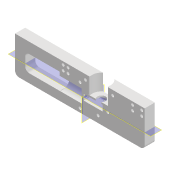
# Autodesk Inventor part: 10_Wellplate_base_p2_v1
Saved by Autodesk Inventor 2022 (Build 260153000, 153)
## iProperties
Created: 2022-04-18
Part Number: 10_Wellplate_base_p2_v1
Material: Generic
Document SubType Name: Modeling
Designer: Prakash Lab
Density: 1 g/cm^3
Appearance: Default
Author: Prakash Lab
Autodesk Inventor part; units mm, degrees
ref_plane "YZ Plane" through (0, 0, 0) normal (1, 0, 0) x (0, 1, 0)
ref_plane "XZ Plane" through (0, 0, 0) normal (0, 1, 0) x (-1, 0, 0)
ref_plane "XY Plane" through (0, 0, 0) normal (0, 0, 1) x (1, 0, 0)
sketch "Sketch1" plane through (0, 0, 0) normal (0, 0, 1) x (1, 0, 0)
  line L0 (63.9, -42.75) -> (-63.9, -42.75)
  line L1 (-63.9, -42.75) -> (-63.9, 0)
  line L2 (-63.9, 0) -> (63.9, 0)
  line L3 (63.9, 0) -> (63.9, -42.75)
  point P0 (0, 0)
  dimension "d0" = 127.8
  dimension "d178" = 63.9
  dimension "d179" = 0
  constraints: 8 end point, 2 parallel, 1 horizontal, 1 perpendicular
  measures "d0" distance of L0.start L0.end
  measures "d178" distance from line of point (0, 0) L1
  measures "d179" distance from line of L2 point (0, 0)
extrude "Extrusion1" add sketch "Sketch1" along normal blind 10
fillet "Fillet1" radius 4 4 edges at (63.9, 0, 5) (-63.9, 0, 5) (-63.9, -42.75, 5) (63.9, -42.75, 5)
sketch "Skizze38" plane through (0, 0, 10) normal (0, 0, 1) x (1, 0, 0)
  line L0 (-63.9, -4) -> (-63.9, -38.75) projected
  arc A0 (-63.9, -38.75) -> (-59.9, -42.75) centre (-59.9, -38.75) ccw projected
  line L1 (-59.9, -42.75) -> (59.9, -42.75) projected
  arc A1 (59.9, -42.75) -> (63.9, -38.75) centre (59.9, -38.75) ccw projected
  line L2 (63.9, -38.75) -> (63.9, -4) projected
  arc A2 (63.9, -4) -> (59.9, 0) centre (59.9, -4) ccw projected
  line L3 (59.9, 0) -> (-59.9, 0) projected
  arc A3 (-59.9, 0) -> (-63.9, -4) centre (-59.9, -4) ccw projected
  point P0 (0, 0)
  point P1 (9.5347, -23.74)
  point P2 (0.0978, -16.7743)
  point P3 (0.0978, -39.0171)
  point P4 (17.95, -36.25)
  point P5 (27.4914, -28.65)
  point P6 (5.4922, -12.0867)
  point P7 (32.285, -12.0867)
hole "Bohrung2" at (0.0978, -16.7743, 10) at (0.0978, -39.0171, 10) at (17.95, -36.25, 10) at (27.4914, -28.65, 10) at (5.4922, -12.0867, 10) at (32.285, -12.0867, 10) direction (0, 0, -1) diameter 2.8 end through all
sketch "Skizze39" plane through (0, 0, 10) normal (0, 0, 1) x (1, 0, 0)
  circle A0 centre (5.4922, -12.0867) radius 1.4 projected
  circle A1 centre (0.0978, -16.7743) radius 1.4 projected
  circle A2 centre (0.0978, -39.0171) radius 1.4 projected
  circle A3 centre (32.285, -12.0867) radius 1.4 projected
  line L0 (-63.9, -4) -> (-63.9, -38.75) projected
  arc A4 (-63.9, -38.75) -> (-59.9, -42.75) centre (-59.9, -38.75) ccw projected
  line L1 (-59.9, -42.75) -> (59.9, -42.75) projected
  arc A5 (59.9, -42.75) -> (63.9, -38.75) centre (59.9, -38.75) ccw projected
  line L2 (63.9, -38.75) -> (63.9, -4) projected
  arc A6 (63.9, -4) -> (59.9, 0) centre (59.9, -4) ccw projected
  line L3 (59.9, 0) -> (-59.9, 0) projected
  arc A7 (-59.9, 0) -> (-63.9, -4) centre (-59.9, -4) ccw projected
  line L4 (63.9, -38.75) -> (63.9, -4) projected
  line L5 (63.9, -7.25) -> (-65.3546, -7.25)
  line L6 (-65.3546, -7.25) -> (-65.3546, -46.5164)
  line L7 (-65.3546, -46.5164) -> (63.9, -46.5164)
  line L8 (63.9, -46.5164) -> (63.9, -7.25)
  point P0 (0, 0)
  point P1 (63.9, 3.9837)
  point P2 (63.9, 14.5163)
  constraints: 8 end point, 2 parallel, 1 horizontal, 1 perpendicular, 1 point on line
extrude "Extrusion36" cut sketch "Skizze39" along normal through all both and the other way through all contours A0 | A1 | A2 | A3 | L5 L2 A5 L1 A4 L0 | L0 A4 L1 A5 L8 L7 L6 L5 keep common part
sketch "Skizze40" plane through (0, 0, 10) normal (0, 0, 1) x (1, 0, 0)
  circle A0 centre (-11.715, -4.25) radius 1.4 projected
  circle A1 centre (-11.715, 0.75) radius 1.4 projected
  circle A2 centre (-16.453, 0.75) radius 1.4 projected
  circle A3 centre (-16.453, -4.25) radius 1.4 projected
  circle A4 centre (51.9, -4.25) radius 1.4 projected
  circle A5 centre (51.9, 0.75) radius 1.4 projected
  circle A6 centre (60.9, 0.75) radius 1.4 projected
  circle A7 centre (60.9, -4.25) radius 1.4 projected
  line L0 (45.9, -7.25) -> (63.9, -7.25) projected
  circle A8 centre (-11.715, -10.25) radius 1.4
  circle A9 centre (-11.715, -15.25) radius 1.4
  circle A10 centre (-16.453, -15.25) radius 1.4
  circle A11 centre (-16.453, -10.25) radius 1.4
  circle A12 centre (51.9, -10.25) radius 1.4
  circle A13 centre (51.9, -15.25) radius 1.4
  circle A14 centre (60.9, -15.25) radius 1.4
  circle A15 centre (60.9, -10.25) radius 1.4
  point P0 (0, 0)
  point P1 (0, -14.5)
  constraints: 9 symmetric about line, 8 centre point, 8 other
extrude "Extrusion37" cut sketch "Skizze40" against normal through all contours A8 | A9 | A10 | A11 | A12 | A13 | A14 | A15
ref_plane "Arbeitsebene10" through (-8.36, -27.75, 5.1474) normal (0, -1, 0) x (1, 0, 0)
sketch "Skizze42" plane through (0, 0, 10) normal (0, 0, 1) x (1, 0, 0)
  line L0 (-63.9, -7.25) -> (-63.9, -38.75) projected
  arc A0 (-63.9, -38.75) -> (-59.9, -42.75) centre (-59.9, -38.75) ccw projected
  line L1 (-59.9, -42.75) -> (59.9, -42.75) projected
  arc A1 (59.9, -42.75) -> (63.9, -38.75) centre (59.9, -38.75) ccw projected
  line L2 (63.9, -38.75) -> (63.9, -7.25) projected
  line L3 (-63.9, -7.25) -> (63.9, -7.25) projected
  circle A2 centre (-11.715, -10.25) radius 1.4 projected
  circle A3 centre (60.9, -10.25) radius 1.4 projected
  circle A4 centre (51.9, -15.25) radius 1.4 projected
  circle A5 centre (-16.453, -15.25) radius 1.4 projected
  circle A6 centre (-11.715, -15.25) radius 1.4 projected
  circle A7 centre (60.9, -15.25) radius 1.4 projected
  circle A8 centre (51.9, -10.25) radius 1.4 projected
  circle A9 centre (-16.453, -10.25) radius 1.4 projected
  circle A10 centre (5.4922, -12.0867) radius 1.4 projected
  circle A11 centre (17.95, -36.25) radius 1.4 projected
  circle A12 centre (0.0978, -16.7743) radius 1.4 projected
  circle A13 centre (0.0978, -39.0171) radius 1.4 projected
  circle A14 centre (27.4914, -28.65) radius 1.4 projected
  circle A15 centre (32.285, -12.0867) radius 1.4 projected
  line L4 (-63.9, -42.75) -> (-19.9, -42.75)
  line L5 (-19.9, -42.75) -> (-19.9, -17.75)
  line L6 (-19.9, -17.75) -> (-63.9, -17.75)
  line L7 (-63.9, -17.75) -> (-63.9, -42.75)
  line L8 (-63.9, -42.75) -> (-53.9, -42.75)
  line L9 (-53.9, -42.75) -> (-53.9, -17.75)
  line L10 (-53.9, -17.75) -> (-63.9, -17.75)
  line L11 (-63.9, -17.75) -> (-63.9, -42.75)
  line L12 (-19.9, -17.75) -> (-53.9, -17.75)
  line L13 (-53.9, -17.75) -> (-53.9, -34.1811)
  line L14 (-53.9, -34.1811) -> (-19.9, -34.1811)
  line L15 (-19.9, -34.1811) -> (-19.9, -17.75)
  point P0 (0, 0)
  point P1 (-63.9, -17.75)
  dimension "d185" = 44
  dimension "d186" = 25
  dimension "d199" = 10
  constraints: 24 end point, 6 parallel, 3 horizontal, 3 perpendicular, 2 point on line
  measures "d185" distance of L6.end L5.end
  measures "d186" distance of L5.end L4.end
  measures "d199" distance of L10.end L9.end
extrude "Extrusion39" cut sketch "Skizze42" against normal blind 66.8 contours A0 L4 L7 | L6 L5 L14 L9
fillet "Rundung7" radius 4 2 edges at (-53.9, -17.75, 5) (-53.9, -34.1811, 5)
sketch "Skizze43" plane through (0, 0, 10) normal (0, 0, 1) x (1, 0, 0)
  line L0 (3.9, -30.55) -> (22.4, -30.55) projected
  line L1 (22.4, -30.55) -> (22.4, -24.95) projected
  line L2 (3.9, -24.95) -> (22.4, -24.95) projected
  line L3 (3.9, -30.55) -> (3.9, -24.95) projected
  line L4 (22.5, -24.85) -> (22.5, -30.65)
  line L5 (22.5, -30.65) -> (3.8, -30.65)
  line L6 (3.8, -30.65) -> (3.8, -24.85)
  line L7 (3.8, -24.85) -> (22.5, -24.85)
  point P0 (0, 0)
  dimension "d190" = 0.1
  constraints: 8 end point, 3 other
  measures "d190" distance between parallel lines of L2 L7
ref_plane "Arbeitsebene11" through (3.9, -30.55, 0.325) normal (0, 0, -1) x (0, 1, 0)
extrude "Extrusion40" cut sketch "Skizze43" against normal up to surface (9.675 mm away) contours L3 L2 L1 L0 | L4 L5 L6 L7
ref_plane "Arbeitsebene14" through (2.9, -38.75, 0) normal (-1, 0, 0) x (0, 0, 1)
sketch "Skizze44" plane through (2.9, -38.75, 0) normal (-1, 0, 0) x (0, 0, 1)
  arc A0 (10.5985, 12.016) -> (10.5985, 9.984) centre (7.125, 11) ccw projected
  circle A1 centre (7.125, 11) radius 2.3038
  point P0 (0, 38.75)
  constraints: 1 centre point, 1 coincident
extrude "Extrusion41" cut sketch "Skizze44" along normal mid plane 10
sketch "Skizze45" plane through (-63.9, -7.25, 10) normal (0, 1, 0) x (1, 0, 0)
  arc A0 (75.7432, 2.4317) -> (78.6377, -2.5817) centre (82.3, 2.875) ccw projected
  line L0 (75.7432, 2.4317) -> (75.545, 2.775) projected
  arc A1 (75.2013, 6) -> (75.545, 2.775) centre (79.0091, 4.775) ccw projected
  line L1 (75.2013, 6) -> (56.8, 6) projected
  line L2 (56.8, -8) -> (56.8, 6) projected
  line L3 (54.8, -8) -> (56.8, -8) projected
  line L4 (54.8, -8) -> (54.8, -18) projected
  line L5 (109.8, -18) -> (54.8, -18) projected
  line L6 (109.8, -8) -> (109.8, -18) projected
  line L7 (107.8, -8) -> (109.8, -8) projected
  line L8 (107.8, -8) -> (107.8, 6) projected
  line L9 (107.8, 6) -> (89.3987, 6) projected
  arc A2 (89.055, 2.775) -> (89.3987, 6) centre (85.5909, 4.775) ccw projected
  line L10 (89.055, 2.775) -> (88.8568, 2.4317) projected
  arc A3 (85.9623, -2.5817) -> (88.8568, 2.4317) centre (82.3, 2.875) ccw projected
  line L11 (85.9623, -2.5817) -> (85.7641, -2.925) projected
  arc A4 (78.8359, -2.925) -> (85.7641, -2.925) centre (82.3, -0.925) ccw projected
  line L12 (78.8359, -2.925) -> (78.6377, -2.5817) projected
  line L13 (127.8, 10) -> (0, 10) projected
  line L14 (0, 10) -> (0, 0) projected
  line L15 (0, 0) -> (127.8, 0) projected
  line L16 (127.8, 0) -> (127.8, 10) projected
  circle A5 centre (82.3, 2.875) radius 7 projected
  circle A6 centre (82.3, 2.875) radius 9
  point P0 (63.9, 10)
  dimension "d197" = 18
  constraints: 1 centre point, 1 coincident
  measures "d197" diameter of A6
ref_plane "Arbeitsebene12" through (3.9, -24.95, 0.325) normal (0, 1, 0) x (0, 0, 1)
extrude "Extrusion42" cut sketch "Skizze45" against normal blind 16 contours L0 A1 A5 A2 L10 A3 L15 A0 | A0 L15 A5 A1 L0 | L15 A3 L11 A4 A5 L12 A0 | A0 L12 A4 A5 L15 | A5 A4 L15 A6 | L15 A6 L1 A1 A5 | L15 A5 A4 L11 A3 | A3 L10 A2 A5 L15 | A1 L1 A6 L13 L9 A2 A5 | A5 A4 | A5 A2 L9 A6 L15 | A6 L13
fillet "Rundung8" radius 1 2 edges at (9.8716, -15.25, 10) (26.9284, -15.25, 10)
sketch "Skizze47" plane through (-63.9, -23.25, 10) normal (0, 1, 0) x (1, 0, 0)
  circle A0 centre (82.3, 2.875) radius 6 projected
  circle A1 centre (82.3, 2.875) radius 4
  point P0 (63.9, 10)
  dimension "d204" = 8
  constraints: 1 centre point, 1 coincident
  measures "d204" diameter of A1
ref_plane "Arbeitsebene13" through (2.975, -27.75, -0.355) normal (0, -1, 0) x (1, 0, 0)
extrude "Extrusion44" cut sketch "Skizze47" against normal up to surface (4.5 mm away) contours A1
sketch "Skizze48" plane through (-19.9, -38.75, 10) normal (-1, 0, 0) x (0, 0, 1)
  circle A0 centre (-2.875, 11) radius 6.7945 projected
  circle A1 centre (-2.875, 11) radius 7.0445
  point P0 (-10, 38.75)
  dimension "d207" = 0.25
  constraints: 1 centre point
  measures "d207" radial gap between concentric circles of A0 A1
ref_plane "Arbeitsebene15" through (1.9, -34.5445, 0.3305) normal (1, 0, 0) x (0, 1, 0)
extrude "Extrusion45" cut sketch "Skizze48" against normal up to surface (21.8 mm away) contours A0 | A1
sketch "Skizze49" plane through (3.8, -30.65, 0.325) normal (0, 0, 1) x (1, 0, 0)
  line L0 (0.1, 0.1) -> (18.6, 0.1) projected
  line L1 (18.6, 0.1) -> (18.6, 5.7) projected
  line L2 (0.1, 5.7) -> (18.6, 5.7) projected
  line L3 (0.1, 0.1) -> (0.1, 5.7) projected
  line L4 (0, 5.8) -> (0, 0) projected
  line L5 (18.7, 0) -> (18.7, 5.8) projected
  line L6 (0, 0) -> (18.7, 0)
  line L7 (18.7, 0) -> (18.7, 1.0978)
  line L8 (18.7, 1.0978) -> (0, 1.0978)
  line L9 (0, 1.0978) -> (0, 0)
  point P0 (-3.8, 30.65)
  point P1 (18.6, 1.0978)
  point P2 (0.1, 1.0978)
  constraints: 8 end point, 2 parallel, 1 horizontal, 1 perpendicular, 1 point on line
extrude "Extrusion46" cut sketch "Skizze49" against normal blind 10 contours L3 L8 L1 L0
body "Solid1"
